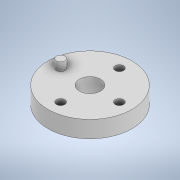
# Autodesk Inventor part: fixhelper
Saved by Autodesk Inventor 2020.3 (Build 243373000, 373)
## iProperties
Created: 2020-10-17
Part Number: fixhelper
Material: 常规
Document SubType Name: Modeling
Designer: Lorne
Density: 1 g/cm^3
Appearance: 默认
Author: Lorne
Autodesk Inventor part; units mm, degrees
ref_plane "YZ Plane" through (0, 0, 0) normal (1, 0, 0) x (0, 1, 0)
ref_plane "XZ Plane" through (0, 0, 0) normal (0, 1, 0) x (-1, 0, 0)
ref_plane "XY Plane" through (0, 0, 0) normal (0, 0, 1) x (1, 0, 0)
sketch "Sketch1" plane through (0, 0, 0) normal (0, 1, 0) x (-1, 0, 0)
  circle A0 centre (0, 0) radius 7
  circle A1 centre (7, 0) radius 1
  circle A2 centre (0, 7) radius 1
  circle A3 centre (-7, 0) radius 1
  circle A4 centre (0, -7) radius 1
  circle A5 centre (0, 0) radius 10
  circle A6 centre (0, 0) radius 2.5
  dimension "d0" = 14
  dimension "d1" = 2
  dimension "d4" = 360
  dimension "d6" = 3
  dimension "d7" = 5
  constraints: 6 centre point, 3 coincident, 1 horizontal alignment, 11 other
  measures "d1" diameter of A1
  measures "d7" diameter of A6
extrude "Extrusion1" add sketch "Sketch1" along normal blind 4 contours A1 A0 A4 A3 A2 | A5
extrude "Extrusion2" add sketch "Sketch1" along normal blind 6 contours A0 A1 | A0 A1
body "Solid1"
